check_siphon_valvemk2 (Autodesk Fusion 360 design; units mm, degrees)
Autodesk Fusion 360 part; units mm, degrees
sketch "Sketch1" plane through (0, 0, 0) normal (0, 0, 1) x (1, 0, 0)
  line L0 (0, 0) -> (0, 100)
  line L1 (-16, 0) -> (-12, 6.9282)
  line L2 (-12, 6.9282) -> (-20, 11.547)
  line L3 (-20, 11.547) -> (-20, 43)
  line L4 (-20, 43) -> (-5.5, 97.1147)
  line L5 (-16, 0) -> (-24, 0)
  line L6 (-24, 0) -> (-24, 60)
  line L7 (-24, 60) -> (-16.5, 66)
  line L8 (-16.5, 66) -> (-8, 66)
  line L9 (-8, 66) -> (-8, 81)
  line L10 (-5.5, 97.1147) -> (-5.5, 81)
  line L11 (-5.5, 81) -> (-8, 81)
  line L12 (0, 0) -> (-16, 0)
  line L13 (-8, 66) -> (-24, 6.2872)
  dimension "d1" = 100
  dimension "d2" = 60
  dimension "d3" = 12
  dimension "d4" = 8
  dimension "d5" = 4
  dimension "d7" = 16
  dimension "d8" = 60
  dimension "d9" = 6
  dimension "d10" = 7.5
  dimension "d12" = 15
  dimension "d13" = 17
  dimension "d14" = 8
  dimension "d15" = 2.5
  dimension "d16" = 8.5
  dimension "d17" = 15
  constraint coincident L0.start L12.start
  constraint vertical L0
  constraint perpendicular L1 L2
  constraint vertical L3
  constraint perpendicular L0 L5
  constraint perpendicular L5 L6
  constraint perpendicular L8 L9
  constraint parallel L11 L12
  constraint parallel L5 L12
  constraint parallel L9 L10
  constraint coincident L6 L13.end
  constraint parallel L4 L13
  measures "d1" distance of L0.start L0.end
  measures "d2" angle of L1 L12
  measures "d3" distance of L0 L1.end
  measures "d4" distance of L1.end L3
  measures "d5" distance of L3 L6
  measures "d7" distance of L0.start L1.start
  measures "d8" distance of L5.end L6.end
  measures "d9" vertical distance of L6.end L7.end
  measures "d10" horizontal distance of L6.end L7.end
  measures "d12" angle of L3 L4
  measures "d13" vertical distance of L3.end L6.end
  measures "d14" distance of L0 L9.end
  measures "d15" distance of L9.end L10.end
  measures "d16" distance of L7.end L8.end
  measures "d17" distance of L8.end L9.end
revolve "Revolve1" add sketch "Sketch1" angle 360 about axis through (0, 0, 0) along (0, 1, 0) contours L1 L2 L3 L5 L6 L13 | L3 L4 L6 L7 L8 L13 makes body 1
sketch "Sketch2" plane through (0, 0, 0) normal (0, 0, 1) x (1, 0, 0)
  line L0 (0, 12) -> (-11, 12)
  line L1 (0, 0) -> (0, 100)
  line L2 (-11, 12) -> (-14.8105, 14.2)
  line L3 (0, 12) -> (0, 47)
  line L4 (-12, 6.9282) -> (-20, 11.547)
  line L5 (-14.8105, 14.2) -> (-14.8105, 15.7)
  line L6 (-14.8105, 15.7) -> (-3, 15.7)
  line L7 (-3, 47) -> (-3, 15.7)
  line L8 (0, 47) -> (-3, 47)
  line L9 (-14.8105, 15.7) -> (-3, 32.7)
  line L10 (-3, 32.7) -> (0, 34.9)
  dimension "d19" = 11
  dimension "d21" = 12
  dimension "d23" = 2.2
  dimension "d24" = 1.5
  dimension "d26" = 3
  dimension "d33" = 35
  dimension "d35" = 17
  dimension "d43" = 2.2
  constraint horizontal L0
  constraint coincident L0.start L1
  constraint coincident L1 L3.end
  constraint parallel L2 L4
  constraint perpendicular L6 L7
  constraint parallel L0 L6
  constraint parallel L1 L5
  constraint perpendicular L1 L8
  constraint coincident L7.start L8.end
  constraint coincident L7 L9.end
  constraint coincident L1 L10.end
  measures "d19" distance of L0.start L0.end
  measures "d21" distance of L0 L1.start
  measures "d23" vertical distance of L0.end L2.end
  measures "d24" distance of L2.end L5.end
  measures "d26" distance of L3 L7
  measures "d33" distance of L0.start L3.end
  measures "d35" distance of L6 L9.end
  measures "d43" vertical distance of L9.end L10.end
sketch "Sketch3" plane through (0, 0, 0) normal (0, 0, 1) x (1, 0, 0)
  line L0 (-20, 11.547) -> (-3.8, 34.8652)
  line L1 (-3.8, 34.8652) -> (-3.8, 35.547)
  line L2 (-3.8, 35.547) -> (-6.8, 35.547)
  line L3 (-6.8, 35.547) -> (-20, 16.547)
  line L4 (-20, 11.547) -> (-20, 43)
  line L5 (-20, 16.547) -> (-20, 11.547)
  line L6 (-3, 47) -> (-3, 15.7)
  line L7 (-14.8105, 15.7) -> (-3, 32.7)
  line L8 (-6.8, 35.547) -> (-6.8, 43.6906)
  line L9 (-6.8, 43.6906) -> (-3.8, 43.6906)
  line L10 (-3.8, 43.6906) -> (-3.8, 35.547)
  dimension "d30" = 5
  dimension "d31" = 3
  dimension "d32" = 0.8
  constraint vertical L1
  constraint perpendicular L1 L2
  constraint parallel L0 L3
  constraint coincident L3.end L4
  constraint coincident L0.start L4
  constraint coincident L0.start L4.start
  constraint parallel L0 L7
  constraint perpendicular L2 L8
  constraint perpendicular L8 L9
  measures "d30" distance of L0.start L3.end
  measures "d31" distance of L1.end L2.end
  measures "d32" distance of L1 L6
revolve "Revolve2" add sketch "Sketch2" angle 360 about axis through (0, 0, 0) along (0, 1, 0) separate body contours L0 L1 L2 L3 L5 L6 L7 L10 | L6 L7 L9 makes body 2
revolve "Revolve3" add sketch "Sketch3" angle 12 about axis through (0, 0, 0) along (0, 1, 0) second angle 12 separate body makes body 3
pattern_circular "C-Pattern1" count 5 over 360 about axis through (0, 0, 0) along (0, 1, 0) of "Revolve3" makes body 4 makes body 5 makes body 6 makes body 7
revolve "Revolve4" add sketch "Sketch3" angle 360 about axis through (0, 0, 0) along (0, 1, 0) contours L2 L8 L9 L10 bodies 3 4 5 6 7
